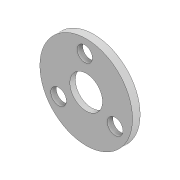
# Autodesk Inventor part: Inner disc of housing of gearbox
Saved by Autodesk Inventor 2020.3 (Build 243373010, 373A)
## iProperties
Created: 2021-05-05
Part Number: Inner disc of housing of gearbox
Material: Generic
Document SubType Name: Modeling
Designer: marti
Density: 1 g/cm^3
Appearance: Default
Author: marti
Autodesk Inventor part; units mm, degrees
ref_plane "YZ Plane" through (0, 0, 0) normal (1, 0, 0) x (0, 1, 0)
ref_plane "XZ Plane" through (0, 0, 0) normal (0, 1, 0) x (-1, 0, 0)
ref_plane "XY Plane" through (0, 0, 0) normal (0, 0, 1) x (1, 0, 0)
sketch "Sketch1" plane through (0, 0, 0) normal (0, 0, 1) x (1, 0, 0)
  circle A0 centre (13.2988, -6.9384) radius 3.6
  circle A1 centre (-12.6582, -8.0479) radius 3.6
  circle A2 centre (-0.6406, 14.9863) radius 3.5
  circle A3 centre (0, 0) radius 7.5
  circle A4 centre (0, 0) radius 21.25
  point P0 (0, 0)
  dimension "d11" = 42.5
  constraints: 5 centre point, 1 coincident
  measures "d11" diameter of A4
extrude "Extrusion1" add sketch "Sketch1" along normal blind 3.5
sketch "Sketch3" plane through (0, 0, 0) normal (0, 0, -1) x (-1, 0, 0)
  circle A0 centre (0, 0) radius 20.25
  dimension "d14" = 40.5
  constraints: 1 centre point, 1 coincident
  measures "d14" diameter of A0
extrude "Extrusion4" cut sketch "Sketch3" against normal blind 1
body "Solid1"
